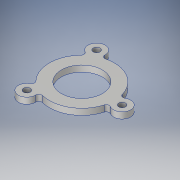
# Autodesk Inventor part: 775 Mounting plate
Saved by Autodesk Inventor 2019.4 (Build 234330000, 330)
## iProperties
Created: 2019-11-30
Part Number: 775 Mounting plate
Material: Aluminum 6061
Document SubType Name: Modeling
Designer: admin
Density: 2.7 g/cm^3
Appearance: Aluminum - Flat
Author: admin
Autodesk Inventor part; units mm, degrees
ref_plane "YZ Plane" through (0, 0, 0) normal (1, 0, 0) x (0, 1, 0)
ref_plane "XZ Plane" through (0, 0, 0) normal (0, 1, 0) x (-1, 0, 0)
ref_plane "XY Plane" through (0, 0, 0) normal (0, 0, 1) x (1, 0, 0)
sketch "Sketch1" plane through (0, 0, 0) normal (0, 1, 0) x (-1, 0, 0)
  circle A0 centre (0, 0) radius 21
  dimension "d0" = 42
  constraints: 1 centre point, 1 coincident
  measures "d0" diameter of A0
extrude "Extrusion1" add sketch "Sketch1" along normal blind 4
sketch "Sketch2" plane through (0, 4, 0) normal (0, 1, 0) x (1, 0, 0)
  circle A0 centre (0, 0) radius 21 projected
  constraints: 1 coincident
hole "Hole1" at (0, 4, 0) direction (0, -1, 0) diameter 26.5 end through all
sketch "Sketch3" plane through (0, 4, 0) normal (0, 1, 0) x (1, 0, 0)
  circle A0 centre (26, 0) radius 2.2
  line L0 (26, 0) -> (0, 0) construction
  circle A1 centre (26, 0) radius 5.5
  circle A2 centre (0, 0) radius 21 projected
  circle A3 centre (-13, 22.5167) radius 2.2
  circle A4 centre (-13, 22.5167) radius 5.5
  circle A5 centre (-13, -22.5167) radius 2.2
  circle A6 centre (-13, -22.5167) radius 5.5
  dimension "d10" = 4.4
  dimension "d11" = 11
  dimension "d14" = 360
  dimension "d19" = 26
  constraints: 6 centre point, 3 coincident, 2 end point, 1 horizontal, 13 other
  measures "d10" diameter of A0
  measures "d11" diameter of A1
  measures "d19" distance of L0.start L0.end
extrude "Extrusion2" add sketch "Sketch3" against normal blind 4 contours A1 A2 | A2 A1 | A4 A2 | A2 A4 | A6 A2 | A2 A6
fillet "Fillet1" radius 2 6 edges at (20.899, 2, -2.0567) (20.899, 2, 2.0567) (-8.6683, 2, 19.1275) (-12.2307, 2, 17.0707) (-12.2307, 2, -17.0707) (-8.6683, 2, -19.1275)
body "Solid1"
